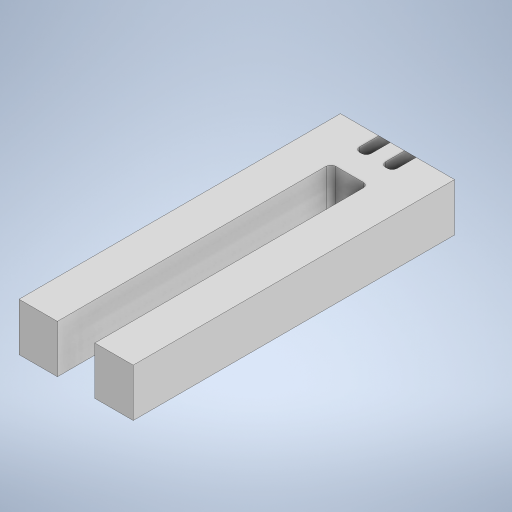
# Autodesk Inventor part: adjuster grip
Saved by Autodesk Inventor 2024 (Build 280153000, 153)
## iProperties
Created: 2025-01-15
Part Number: adjuster grip
Material: Generic
Document SubType Name: Modeling
Designer: Williamow
Density: 1 g/cm^3
Appearance: Default
Author: Williamow
Autodesk Inventor part; units mm, degrees
ref_plane "YZ Plane" through (0, 0, 0) normal (1, 0, 0) x (0, 1, 0)
ref_plane "XZ Plane" through (0, 0, 0) normal (0, 1, 0) x (-1, 0, 0)
ref_plane "XY Plane" through (0, 0, 0) normal (0, 0, 1) x (1, 0, 0)
sketch "Sketch1" plane through (0, 0, 0) normal (0, 1, 0) x (-1, 0, 0)
  line L0 (-1.5, 5) -> (-1.5, -13)
  line L1 (-1.5, -13) -> (0, -13)
  line L2 (0, -13) -> (0, 0)
  line L3 (0, 0) -> (2.4, 0)
  line L4 (2.4, 0) -> (2.4, -10)
  line L5 (2.4, -10) -> (0.4, -10)
  line L6 (0.4, -10) -> (0.4, -13)
  line L7 (0.4, -13) -> (10.4, -13)
  line L8 (10.4, -13) -> (10.4, 62)
  line L9 (10.4, 62) -> (2.4, 62)
  line L10 (2.4, 62) -> (2.4, 5)
  line L11 (2.4, 5) -> (-1.5, 5)
  dimension "d0" = 0.4
  dimension "d1" = 2
  dimension "d2" = 10
  dimension "d3" = 75
  dimension "d4" = 5
  dimension "d5" = 10
  dimension "d6" = 3
  dimension "d7" = 1.5
  constraints: 24 end point, 9 perpendicular, 4 point on line, 1 coincident, 1 vertical, 1 vertical alignment
  measures "d0" distance of L6.end L1.end
  measures "d1" distance of L4.end L5.end
  measures "d2" distance of L6.end L7.end
  measures "d3" distance of L7.end L8.end
  measures "d4" distance between parallel lines of L3 L11
  measures "d5" distance of L3.end L4.end
  measures "d6" distance of L5.end L6.end
  measures "d7" distance of L0.end L1.end
extrude "Extrusion1" add sketch "Sketch1" along normal blind 10
mirror "Mirror1" about plane through (1.5, 0, 5) normal (1, 0, 0) of "Extrusion1"
chamfer "Chamfer1" distance 8 angle 45 5 edges at (-5.4, 10, -13) (1.5, 10, -13) (8.4, 10, -13) (13.4, 5, -13) (-10.4, 5, -13)
fillet "Fillet1" radius 1 12 edges at (-0.4, 1, -13) (0, 1, -13) (3.4, 1, -13) (3, 1, -13) (-0.4, 2.5, -10) (3.4, 2.5, -10) (5.4, 5, 0) (3, 5, 0) (0, 5, 0) (-2.4, 5, 0) (-2.4, 5, 5) (5.4, 5, 5)
body "Solid1"
